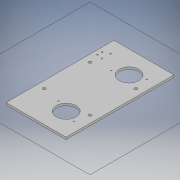
# Autodesk Inventor part: 000.001.006 - Площадка под манипулятор
Saved by Autodesk Inventor 2022 (Build 260153000, 153)
## iProperties
Created: 2022-02-27
Part Number: 000.001.006 - Площадка под манипулятор
Material: Типовые
Document SubType Name: Modeling
Designer: Petrov Ivan
Density: 1 g/cm^3
Appearance: По умолчанию
Author: Petrov Ivan
Autodesk Inventor part; units mm, degrees
ref_plane "YZ Plane" through (0, 0, 0) normal (1, 0, 0) x (0, 1, 0)
ref_plane "XZ Plane" through (0, 0, 0) normal (0, 1, 0) x (-1, 0, 0)
ref_plane "XY Plane" through (0, 0, 0) normal (0, 0, 1) x (1, 0, 0)
sketch "Эскиз1" plane through (0, 0, 0) normal (0, 1, 0) x (-1, 0, 0)
  line L0 (-80, 144) -> (80, 144)
  line L1 (80, 144) -> (80, -144)
  line L2 (80, -144) -> (-80, -144)
  line L3 (-80, -144) -> (-80, 144)
  line L4 (-80, 144) -> (80, -144) construction
  line L5 (80, 144) -> (-80, -144) construction
  point P0 (0, 0)
  dimension "d0" = 160
  dimension "d1" = 288
  constraints: 12 end point, 2 midpoint, 2 parallel, 1 horizontal, 1 perpendicular
  measures "d0" distance of L1.end L2.end
  measures "d1" distance of L0.end L1.end
extrude "Выдавливание1" add sketch "Эскиз1" along normal blind 6
sketch "Эскиз4" plane through (0, 6, 0) normal (0, 1, 0) x (1, 0, 0)
  circle A0 centre (63.6396, 63.6396) radius 4
  line L0 (0, 0) -> (31.2937, 0) construction
  line L1 (63.6396, 63.6396) -> (0, 0) construction
  dimension "d8" = 8
  dimension "d9" = 90
  dimension "d10" = 45
  constraints: 4 end point, 1 centre point, 1 horizontal
  measures "d8" diameter of A0
  measures "d9" distance of L0.start L1.start
  measures "d10" angle of L0 L1
extrude "Выдавливание4" [suppressed]
pattern_circular "Круговой массив1" [suppressed]
sketch "Эскиз6" plane through (0, 0, 0) normal (0, -1, 0) x (1, 0, 0)
  circle A0 centre (-61.251, 61.2502) radius 4 projected
  circle A1 centre (-61.251, -61.2641) radius 4 projected
  circle A2 centre (61.2633, -61.2641) radius 4 projected
  circle A3 centre (61.2633, 61.2502) radius 4 projected
  circle A4 centre (20.3596, -84) radius 26.5 projected
  circle A5 centre (20.3596, 84) radius 26.5 projected
  point P0 (0, 0)
extrude "Выдавливание5" cut sketch "Эскиз6" against normal blind 10
sketch "Эскиз7" plane through (0, 0, 0) normal (0, -1, 0) x (1, 0, 0)
  circle A0 centre (-13.5545, -70.7681) radius 1.5 projected
  circle A1 centre (54.2737, -97.2319) radius 1.5 projected
  circle A2 centre (54.2737, 97.2319) radius 1.5 projected
  circle A3 centre (-13.5545, 70.7681) radius 1.5 projected
  point P0 (0, 0)
extrude "Выдавливание6" cut sketch "Эскиз7" against normal blind 10
sketch "Эскиз8" plane through (0, 0, 0) normal (0, -1, 0) x (1, 0, 0)
  circle A0 centre (-68.825, -100.977) radius 2 projected
  circle A1 centre (-68.825, -88.977) radius 2 projected
  circle A2 centre (-53.825, -86.0186) radius 2 projected
  circle A3 centre (-53.825, -108.4524) radius 2 projected
  point P0 (0, 0)
extrude "Выдавливание7" cut sketch "Эскиз8" against normal blind 10
